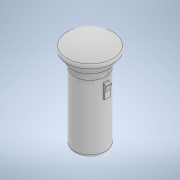
# Autodesk Inventor part: фонарь
Saved by Autodesk Inventor 2021 (Build 250183000, 183)
## iProperties
Created: 2023-01-20
Part Number: фонарь
Material: Типовые
Document SubType Name: Modeling
Designer: Ozornin_NA
Density: 1 g/cm^3
Appearance: По умолчанию
Author: Ozornin_NA
Autodesk Inventor part; units mm, degrees
ref_plane "XZ Plane" through (0, 0, 0) normal (0, 1, 0) x (-1, 0, 0)
ref_plane "XY Plane" through (0, 0, 0) normal (0, 0, 1) x (1, 0, 0)
sketch "Эскиз1" plane through (0, 0, 0) normal (1, 0, 0) x (0, 1, 0)
  line L0 (0, 0) -> (14.8374, 0)
  line L1 (0, 2.439) -> (0, 0)
  line L2 (11.5443, 2.7805) -> (13.0941, 3.8251)
  arc A0 (14.8374, 0) -> (13.0941, 3.8251) centre (9.7692, 0) ccw
  line L3 (13.0941, 3.8251) -> (13.0941, -3.8251) construction
  line L4 (13.0941, 3.8251) -> (20.7443, 3.8251) construction
  line L5 (14.8374, 2.439) -> (14.8374, 0)
  line L6 (14.8374, 2.439) -> (14.2119, 2.439)
  line L7 (10.4265, 2.439) -> (0, 2.439)
  arc A1 (10.4265, 2.439) -> (11.5443, 2.7805) centre (10.4265, 4.439) ccw
  dimension "d2" = 90
  dimension "d3" = 2
  dimension "d7" = 2.439
  dimension "d15" = 14.8374
  constraints: 16 end point, 5 point on circle, 2 centre point, 2 horizontal, 2 parallel, 2 tangent, 1 perpendicular
  measures "d2" angle of L3 L4
  measures "d3" radius of A1
  measures "d7" distance between parallel lines of L7 L0
  measures "d15" distance of L0.start L0.end
revolve "Вращение1" add sketch "Эскиз1" angle 360 about axis through (0, 0, 0) along (0, 1, 0) contours L1 L7 A1 L2 A0 L0
fillet "Сопряжение1" radius 0.5 1 edges at (0, 0, -2.439)
fillet "Сопряжение2" radius 0.5 1 edges at (0, 13.0941, -3.8251)
ref_plane "РабПлоскость1" through (2.439, 0, 0) normal (1, 0, 0) x (0, 1, 0)
sketch "Эскиз2" plane through (2.439, 0, 0) normal (1, 0, 0) x (0, 1, 0)
  point P0 (0, 0)
sketch "Эскиз3" plane through (2.439, 0, 0) normal (1, 0, 0) x (0, 1, 0)
  line L0 (9.7176, 0.4017) -> (7.5973, 0.4017)
  line L1 (7.5973, 0.4017) -> (7.5973, 0)
  line L2 (7.5973, 0) -> (9.7176, 0)
  line L3 (9.7176, 0) -> (9.7176, 0.4017)
  line L4 (9.7176, -0.4017) -> (7.5973, -0.4017)
  line L5 (7.5973, -0.4017) -> (7.5973, 0)
  line L6 (9.7176, 0) -> (9.7176, -0.4017)
  point P0 (0, 0)
  constraints: 14 end point, 2 parallel, 2 symmetric about line, 1 horizontal, 1 perpendicular
extrude "Выдавливание1" add sketch "Эскиз3" along normal blind 0.5 and the other way blind 0.5
sketch "Эскиз4" plane through (2.4057, 7.5973, 0.4017) normal (0, 0, 1) x (1, 0, 0)
  point P0 (-2.4057, -7.5973)
sketch "Эскиз5" plane through (2.4057, 7.5973, 0.4017) normal (0, 0, 1) x (1, 0, 0)
  line L0 (0, 0) -> (0, 2.1203) projected
  line L1 (0, 0) -> (0.5333, 0) projected
  line L2 (0.5333, 2.1203) -> (0.5333, 0) projected
  line L3 (0, 2.1203) -> (0.5333, 2.1203) projected
  line L4 (0, 0) -> (0, 2.1203) projected
  arc A0 (0.546, 1.9689) -> (0, 2.1203) centre (0, 1.0602) ccw
  line L5 (0.5333, 2.1203) -> (0.5333, 0) projected
  arc A1 (0, 0) -> (0.5333, 0.1439) centre (0, 1.0602) ccw
  line L6 (0.546, 1.9689) -> (0.2762, 1.0602)
  line L7 (0.2762, 1.0602) -> (0.2762, 0.0366)
  point P0 (-2.4057, -7.5973)
  point P1 (0.5333, 1.926)
  point P2 (0.5333, 1.9764)
  constraints: 6 point on circle, 4 end point, 2 centre point, 1 coincident, 1 midpoint, 1 point on line
extrude "Выдавливание2" cut sketch "Эскиз5" against normal through all contours A1 L2 L1 | L3 L2 A0 | L7 L6 L2 A1
